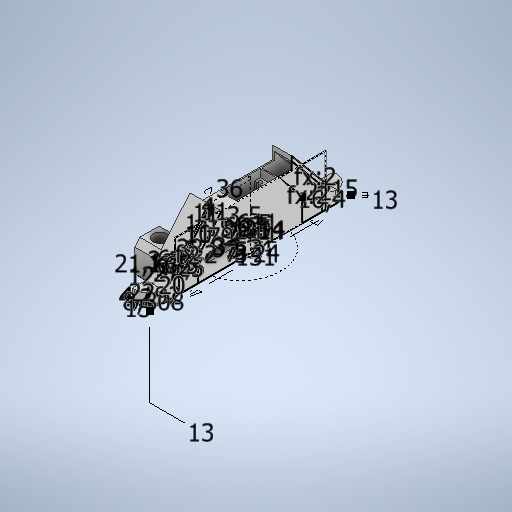
# Autodesk Inventor part: new_back_part
Saved by Autodesk Inventor 2025 (Build 290162000, 162)
## iProperties
Created: 2026-09-04
Part Number: new_back_part
Material: Типовые
Document SubType Name: Modeling
Designer: garin
Density: 1 g/cm^3
Appearance: По умолчанию
Author: garin
Autodesk Inventor part; units mm, degrees
ref_plane "YZ Plane" through (0, 0, 0) normal (1, 0, 0) x (0, 1, 0)
ref_plane "XZ Plane" through (0, 0, 0) normal (0, 1, 0) x (-1, 0, 0)
ref_plane "XY Plane" through (0, 0, 0) normal (0, 0, 1) x (1, 0, 0)
sketch "Эскиз1" plane through (0, 0, 0) normal (0, 1, 0) x (-1, 0, 0)
  line L0 (7, 5) -> (-7, 5)
  line L1 (-7, 5) -> (-7, -19)
  line L2 (-7, -19) -> (7, -19)
  line L3 (7, -19) -> (7, 5)
  line L4 (0, 5) -> (0, 0) construction
  line L5 (-3.5, 3.25) -> (3.5, 3.25) construction
  line L6 (3.5, 3.25) -> (3.5, 6.75) construction
  line L7 (3.5, 6.75) -> (-3.5, 6.75) construction
  line L8 (-3.5, 6.75) -> (-3.5, 3.25) construction
  line L9 (-3.5, 3.25) -> (3.5, 6.75) construction
  line L10 (3.5, 3.25) -> (-3.5, 6.75) construction
  circle A0 centre (3.5, 6.75) radius 1.5
  circle A1 centre (-3.5, 6.75) radius 1.5
  line L11 (2, 6.75) -> (2, 5)
  line L12 (5, 6.75) -> (5, 5)
  line L13 (-2, 6.75) -> (-2, 5)
  line L14 (-5, 6.75) -> (-5, 5)
  line L15 (7, -7) -> (-7, -7) construction
  circle A2 centre (3.5, -20.75) radius 1.5
  circle A3 centre (-3.5, -20.75) radius 1.5
  line L16 (2, -20.75) -> (2, -19)
  line L17 (5, -20.75) -> (5, -19)
  line L18 (-2, -20.75) -> (-2, -19)
  line L19 (-5, -20.75) -> (-5, -19)
  line L20 (0, 0) -> (-8.2, 0) construction
  line L21 (8.2, 65.5) -> (-8.2, 65.5)
  line L22 (-8.2, 65.5) -> (-8.2, -65.5)
  line L23 (-8.2, -65.5) -> (8.2, -65.5)
  line L24 (8.2, -65.5) -> (8.2, 65.5)
  line L25 (-8.2, -65.5) -> (6.8, -65.5)
  line L26 (6.8, -65.5) -> (6.8, -87.5)
  line L27 (6.8, -87.5) -> (4.8, -87.5)
  line L28 (-8.2, -74.5) -> (-8.2, -65.5)
  line L29 (-8.2, 65.5) -> (6.8, 65.5)
  line L30 (6.8, 65.5) -> (6.8, 87.5)
  line L31 (6.8, 87.5) -> (4.8, 87.5)
  line L32 (-8.2, 74.5) -> (-8.2, 65.5)
  arc A4 (4.8, 87.5) -> (-8.2, 74.5) centre (4.8, 74.5) ccw
  arc A5 (-8.2, -74.5) -> (4.8, -87.5) centre (4.8, -74.5) ccw
  circle A6 centre (0, 0) radius 35 construction
  line L33 (24, -5.5) -> (35, -5.5) construction
  line L34 (35, -5.5) -> (35, 5.5) construction
  line L35 (35, 5.5) -> (24, 5.5) construction
  line L36 (24, 5.5) -> (24, -5.5) construction
  line L37 (24, -5.5) -> (34, -5.5) construction
  line L38 (34, -5.5) -> (34, 5.5) construction
  line L39 (34, 5.5) -> (24, 5.5) construction
  line L40 (24, 5.5) -> (24, -5.5) construction
  line L41 (0, 0) -> (35, 0) construction
  line L42 (-5.5, -35) -> (5.5, -35) construction
  line L43 (5.5, -35) -> (5.5, -24) construction
  line L44 (5.5, -24) -> (-5.5, -24) construction
  line L45 (-5.5, -24) -> (-5.5, -35) construction
  line L46 (0, 0) -> (0, -35) construction
  line L47 (7, 10) -> (-7, 10)
  line L48 (-7, 10) -> (-7, -24)
  line L49 (-7, -24) -> (7, -24)
  line L50 (7, -24) -> (7, 10)
  line L51 (7, 10) -> (-7, -24) construction
  line L52 (-7, 10) -> (7, -24) construction
  line L53 (-8.2, 74.5) -> (0.608, 74.5) construction
  line L54 (0.608, 74.5) -> (0.608, 78.692) construction
  line L55 (0.608, 78.692) -> (-8.2, 78.692) construction
  line L56 (-8.2, 78.692) -> (-8.2, 74.5) construction
  circle A7 centre (0.608, 78.692) radius 2.1
  circle A8 centre (0.608, -78.692) radius 2.1
  line L57 (8.2, 0) -> (14.7, 0) construction
  line L58 (14.7, 0) -> (14.7, -19.2) construction
  line L59 (14.7, -19.2) -> (8.2, -19.2) construction
  line L60 (8.2, -19.2) -> (8.2, 0) construction
  circle A9 centre (14.7, -19.2) radius 1.75
  line L61 (8.2, 0) -> (14.7, 0) construction
  line L62 (14.7, 0) -> (14.7, 38.8) construction
  line L63 (14.7, 38.8) -> (8.2, 38.8) construction
  line L64 (8.2, 38.8) -> (8.2, 0) construction
  circle A10 centre (14.7, 38.8) radius 1.75
  line L65 (17.95, -22.45) -> (11.45, -22.45)
  line L66 (11.45, -22.45) -> (11.45, -15.95)
  line L67 (11.45, -15.95) -> (17.95, -15.95)
  line L68 (17.95, -15.95) -> (17.95, -22.45)
  line L69 (17.95, -22.45) -> (11.45, -15.95) construction
  line L70 (11.45, -22.45) -> (17.95, -15.95) construction
  line L71 (11.45, -22.45) -> (8.2, -22.45)
  line L72 (8.2, -22.45) -> (8.2, -15.95)
  line L73 (8.2, -15.95) -> (11.45, -15.95)
  line L74 (11.45, -15.95) -> (11.45, -22.45)
  line L75 (11.45, 35.55) -> (17.95, 35.55)
  line L76 (17.95, 35.55) -> (17.95, 42.05)
  line L77 (17.95, 42.05) -> (11.45, 42.05)
  line L78 (11.45, 42.05) -> (11.45, 35.55)
  line L79 (11.45, 35.55) -> (17.95, 42.05) construction
  line L80 (17.95, 35.55) -> (11.45, 42.05) construction
  line L81 (11.45, 35.55) -> (8.2, 35.55)
  line L82 (8.2, 35.55) -> (8.2, 42.05)
  line L83 (8.2, 42.05) -> (11.45, 42.05)
  line L84 (11.45, 42.05) -> (11.45, 35.55)
  line L85 (8.2, 65.5) -> (26.7, 65.5)
  line L86 (26.7, 65.5) -> (26.7, 44.35)
  line L87 (26.7, 44.35) -> (8.2, 44.35)
  line L88 (8.2, 44.35) -> (8.2, 65.5)
  line L89 (26.7, 54.925) -> (8.2, 54.925) construction
  line L90 (17.45, 65.5) -> (17.45, 44.35) construction
  line L91 (17.95, 42.05) -> (8.2, 42.05)
  line L92 (8.2, 42.05) -> (8.2, 44.35)
  line L93 (8.2, 44.35) -> (17.95, 44.35)
  line L94 (17.95, 44.35) -> (17.95, 42.05)
  line L95 (17.45, 54.925) -> (17.45, 52.925) construction
  circle A11 centre (17.45, 52.925) radius 6
  point P0 (-8.2, -87.5)
  point P1 (-8.2, 87.5)
  point P2 (6.8, -65.5)
  point P3 (6.8, 65.5)
  point P4 (0, -7)
  point P5 (7, 5)
  point P6 (-7, 5)
  point P7 (-7, -19)
  point P8 (8.2, 42.05)
  point P9 (8.2, 35.55)
  point P10 (8.2, -15.95)
  point P11 (8.2, -22.45)
  point P12 (17.95, 44.35)
  point P13 (8.2, 44.35)
  dimension "d0" = 14
  dimension "d1" = 24
  dimension "d2" = 5
  dimension "d3" = 7
  dimension "d4" = 3.5
  dimension "d5" = 3
  dimension "d6" = 3
  dimension "d7" = 8.2
  dimension "d8" = 16.4
  dimension "d9" = 131
  dimension "d10" = 15
  dimension "d11" = 22
  dimension "d12" = 15
  dimension "d13" = 22
  dimension "d14" = 13
  dimension "d15" = 13
  dimension "d24" = 70
  dimension "d25" = 11
  dimension "d26" = 11
  dimension "d27" = 10
  dimension "d28" = 11
  dimension "d29" = 11
  dimension "d32" = 14
  dimension "d33" = 34
  dimension "d77" = 8.808
  dimension "d78" = 4.192
  dimension "d79" = 4.2
  dimension "d82" = 6.5
  dimension "d83" = 19.2
  dimension "d84" = 3.5
  dimension "d85" = 6.5
  dimension "d86" = 38.8
  dimension "d87" = 3.5
  dimension "d88" = 6.5
  dimension "d89" = 6.5
  dimension "d90" = 3.25
  dimension "d91" = 6.5
  dimension "d92" = 6.5
  dimension "d93" = 6.5
  dimension "d94" = 3.25
  dimension "d95" = 6.5
  dimension "d105" = 18.5
  dimension "d106" = 21.15
  dimension "d115" = 2
  dimension "d116" = 12
  constraints: 192 end point, 36 parallel, 24 perpendicular, 21 midpoint, 18 horizontal, 14 point on circle, 14 point on line, 12 centre point, 11 symmetric about line, 8 coincident, 8 tangent, 2 vertical, 3 other
  measures "d0" distance of L2.end L1.end
  measures "d1" distance of L1.end L0.end
  measures "d2" distance of L4.start L4.end
  measures "d3" distance of L7.end L6.end
  measures "d4" distance of L6.end L5.end
  measures "d5" diameter of A0
  measures "d6" diameter of A1
  measures "d7" distance of L20.end L4.end
  measures "d8" distance of L23.end L22.end
  measures "d9" distance of L22.end L21.end
  measures "d10" distance of L26.end point (-8.2, -87.5)
  measures "d11" distance of L25.end L26.end
  measures "d12" distance of point (-8.2, 87.5) L30.end
  measures "d13" distance of L30.end L29.end
  measures "d14" radius of A4
  measures "d15" radius of A5
  measures "d24" diameter of A6
  measures "d25" distance of L35.end L34.end
  measures "d26" distance of L34.end L33.end
  measures "d27" distance of L39.end L38.end
  measures "d28" distance of L44.end L43.end
  measures "d29" distance of L43.end L42.end
  measures "d32" distance of L49.end L48.end
  measures "d33" distance of L48.end L47.end
  measures "d77" distance of L55.end L54.end
  measures "d78" distance of L54.end L53.end
  measures "d79" diameter of A7
  measures "d82" distance of L58.end L59.end
  measures "d83" distance of L57.end L58.end
  measures "d84" diameter of A9
  measures "d85" distance of L63.end L62.end
  measures "d86" distance of L62.end L61.end
  measures "d87" diameter of A10
  measures "d88" distance of L66.end L67.end
  measures "d89" distance of L65.end L66.end
  measures "d90" distance of L72.end L73.end
  measures "d91" distance of L71.end L72.end
  measures "d92" distance of L77.end L76.end
  measures "d93" distance of L76.end L75.end
  measures "d94" distance of L82.end L83.end
  measures "d95" distance of L81.end L82.end
  measures "d105" distance of L86.end L87.end
  measures "d106" distance of L85.end L86.end
  measures "d115" distance of L95.start L95.end
  measures "d116" diameter of A11
extrude "Выдавливание1" add sketch "Эскиз1" along normal blind 44.3 contours L3 L2 L1 L0 | L0 L12 A0 L11 L13 A1 L14 L48 L47 L50 | L0 L11 A0 L12 | L50 L49 L48 L2 L19 A3 L18 L16 A2 L17 | A0 | L17 A2 L16 L2 | L0 L14 A1 L13 | A2 | A1 | L18 A3 L19 L2 | A3 | L24 L23 L22 L21
extrude "Выдавливание2" add sketch "Эскиз1" along normal blind 10 contours L21 L32 A4 L31 L30 | L23 L26 L27 A5 L28 | A7 | A8
extrude "Выдавливание6" cut sketch "Эскиз1" against normal blind 7 from surface at 44.3 contours L3 L2 L1 L0 | L0 L12 A0 L11 L13 A1 L14 L48 L47 L50 | L0 L11 A0 L12 | L50 L49 L48 L2 L19 A3 L18 L16 A2 L17 | A0 | L17 A2 L16 L2 | L0 L14 A1 L13 | A2 | A1 | L18 A3 L19 L2 | A3
extrude "Выдавливание7" cut sketch "Эскиз1" against normal blind 22 from surface at 37.3 contours L3 L2 L1 L0
extrude "Выдавливание8" cut sketch "Эскиз1" against normal blind 6 from surface at 37.3 contours L0 L11 A0 L12 | A0 | L17 A2 L16 L2 | L0 L14 A1 L13 | A2 | A1 | L18 A3 L19 L2 | A3
fillet "Сопряжение1" radius 10 2 edges at (0.7, 10, 65.5) (0.7, 10, -65.5)
sketch "Эскиз4" plane through (8.2, 44.3, 65.5) normal (1, 0, 0) x (0, 0, -1)
  line L0 (131, 0) -> (0, 0) construction
  line L1 (131, -44.3) -> (0, -44.3) construction
  line L2 (0, 0) -> (131, 0) construction
  line L3 (131, 0) -> (131, -44.3) construction
  line L4 (131, -44.3) -> (0, -44.3) construction
  line L5 (0, -44.3) -> (0, 0) construction
  line L6 (65.5, 0) -> (65.5, -44.3) construction
  line L7 (65.5, 0) -> (29.5, 0) construction
  line L8 (29.5, 0) -> (29.5, 11)
  line L9 (29.5, 11) -> (65.5, 11) construction
  line L10 (65.5, 11) -> (65.5, 0) construction
  line L11 (0, -44.3) -> (0, -24.3)
  line L12 (0, -24.3) -> (29.5, 11)
  line L13 (29.5, 0) -> (40.5, 0)
  line L14 (40.5, 0) -> (21.4751, -22.7653)
  line L15 (0, -24.3) -> (20.1926, -24.3) construction
  line L16 (20.1926, -26.3) -> (20.1926, -44.3)
  line L17 (0, -44.3) -> (20.1926, -44.3) construction
  line L18 (29.5, 11) -> (29.5, 7) construction
  line L19 (29.5, 7) -> (3.3428, -24.3)
  line L20 (3.3428, -24.3) -> (3.3428, -44.3)
  line L21 (0, -44.3) -> (20.1926, -44.3)
  line L22 (101.5, 0) -> (101.5, 11)
  line L23 (131, -44.3) -> (131, -24.3)
  line L24 (131, -24.3) -> (101.5, 11)
  line L25 (101.5, 0) -> (90.5, 0)
  line L26 (90.5, 0) -> (109.5249, -22.7653)
  line L27 (110.8074, -26.3) -> (110.8074, -44.3)
  line L28 (101.5, 7) -> (127.6572, -24.3)
  line L29 (127.6572, -24.3) -> (127.6572, -44.3)
  line L30 (131, -44.3) -> (110.8074, -44.3)
  line L31 (20.3074, 0) -> (0, 0)
  line L32 (0, 0) -> (0, -24.3)
  line L33 (110.6926, 0) -> (131, 0)
  line L34 (131, 0) -> (131, -24.3)
  line L35 (21.4751, -22.7653) -> (20.1926, -26.3)
  line L36 (109.5249, -22.7653) -> (110.8074, -26.3)
  point P0 (3.3428, -44.3)
  point P1 (110.8074, -24.3)
  point P2 (127.6572, -44.3)
  point P3 (110.6926, 0)
  dimension "d54" = 36
  dimension "d55" = 11
  dimension "d56" = 20
  dimension "d57" = 11
  dimension "d58" = 4
  dimension "d73" = 2
  dimension "d74" = 2
  dimension "d75" = 2
  dimension "d76" = 2
  constraints: 70 end point, 15 point on line, 11 symmetric about line, 6 parallel, 5 perpendicular, 4 collinear, 2 horizontal, 1 midpoint, 1 vertical
  measures "d54" distance of L8.end L9.end
  measures "d55" distance of L7.end L8.end
  measures "d56" distance of L4.end L11.end
  measures "d57" distance of L7.end L13.end
  measures "d58" distance of L8.end L18.end
  measures "d73" distance of L14.end L15.end
  measures "d74" distance of L16.start L15.end
  measures "d75" distance of L26.end point (110.807, -24.3)
  measures "d76" distance of L27.start point (110.807, -24.3)
ref_plane "РабПлоскость1" through (7, 44.3, 65.5) normal (1, 0, 0) x (0, 0, -1)
ref_plane "РабПлоскость2" through (-7, 0, -65.5) normal (-1, 0, 0) x (0, 0, 1)
extrude "Выдавливание9" cut sketch "Эскиз4" against normal blind 14 from surface at -1.2 contours L13 L14 L35 L16 L21 L20 L19 L8 | L22 L28 L29 L30 L27 L36 L26 L25 | L22 L24 L23 L30 L29 L28
extrude "Выдавливание10" add sketch "Эскиз4" against normal blind 16.4 contours L19 L20 L21 L11 L12 L8 | L22 L24 L23 L30 L29 L28
extrude "Выдавливание11" cut sketch "Эскиз4" against normal blind 16.4 contours L12 L32 L31 | L33 L34 L24
extrude "Выдавливание12" add sketch "Эскиз4" against normal blind 1.2 contours L13 L14 L35 L16 L21 L20 L19 L8 | L22 L28 L29 L30 L27 L36 L26 L25 | L22 L24 L23 L30 L29 L28
extrude "Выдавливание13" add sketch "Эскиз4" along normal blind 1.2 from surface at -16.4 contours L13 L14 L35 L16 L21 L20 L19 L8 | L22 L28 L29 L30 L27 L36 L26 L25 | L22 L24 L23 L30 L29 L28
fillet "Сопряжение2" radius 2 2 edges at (-6.8, 10, 65.5) (-6.8, 10, -65.5)
fillet "Сопряжение3" radius 1 1 edges at (0, 44.3, 10)
extrude "Выдавливание14" cut sketch "Эскиз1" along normal blind 6 contours A7 | A8
extrude "Выдавливание15" add sketch "Эскиз1" along normal blind 11.6 contours L87 L94 L77 L83 L24 | L83 L78 L81 L24 | L77 L76 L75 L78 | L73 L66 L71 L24 | L67 L68 L65 L66 | A9 | A10
fillet "Сопряжение4" radius 2 6 edges at (-17.95, 5.8, -22.45) (-8.2, 5.8, -22.45) (-8.2, 5.8, -15.95) (-17.95, 5.8, -15.95) (-17.95, 5.8, 35.55) (-8.2, 5.8, 35.55)
extrude "Выдавливание16" cut sketch "Эскиз1" against normal blind 6 from surface at 11.6 contours A9 | A10
sketch "Эскиз6" plane through (-8.2, 44.3, 36) normal (-1, 0, 0) x (0, 0, 1)
  line L0 (0.6, -29.4) -> (0.6, -28.84) projected
  arc A0 (-0.7, -30.7) -> (0.6, -29.4) centre (-0.7, -29.4) ccw projected
  line L1 (-0.7, -30.7) -> (-7.04, -30.7) projected
  arc A1 (-8.34, -29.4) -> (-7.04, -30.7) centre (-7.04, -29.4) ccw projected
  line L2 (-8.34, -29.4) -> (-8.34, -28.84) projected
  arc A2 (-7.04, -27.54) -> (-8.34, -28.84) centre (-7.04, -28.84) ccw projected
  line L3 (-0.7, -27.54) -> (-7.04, -27.54) projected
  arc A3 (0.6, -28.84) -> (-0.7, -27.54) centre (-0.7, -28.84) ccw projected
  arc A4 (-7.04, -27.84) -> (-8.04, -28.84) centre (-7.04, -28.84) ccw projected
  line L4 (-8.04, -29.4) -> (-8.04, -28.84) projected
  arc A5 (-8.04, -29.4) -> (-7.04, -30.4) centre (-7.04, -29.4) ccw projected
  line L5 (-7.04, -30.4) -> (-0.7, -30.4) projected
  arc A6 (-0.7, -30.4) -> (0.3, -29.4) centre (-0.7, -29.4) ccw projected
  line L6 (0.3, -28.84) -> (0.3, -29.4) projected
  arc A7 (0.3, -28.84) -> (-0.7, -27.84) centre (-0.7, -28.84) ccw projected
  line L7 (-0.7, -27.84) -> (-7.04, -27.84) projected
  arc A8 (-7.04, -25.54) -> (-10.34, -28.84) centre (-7.04, -28.84) ccw construction
  line L8 (-10.34, -28.84) -> (-10.34, -29.4) construction
  arc A9 (-10.34, -29.4) -> (-7.04, -32.7) centre (-7.04, -29.4) ccw construction
  line L9 (-7.04, -32.7) -> (-0.7, -32.7) construction
  arc A10 (-0.7, -32.7) -> (2.6, -29.4) centre (-0.7, -29.4) ccw
  line L10 (2.6, -29.4) -> (2.6, -28.84)
  arc A11 (2.6, -28.84) -> (-0.7, -25.54) centre (-0.7, -28.84) ccw
  line L11 (-0.7, -25.54) -> (-7.04, -25.54) construction
  line L12 (-15.7, -27.8) -> (-21.3, -27.8) projected
  arc A12 (-15.25, -28.25) -> (-15.7, -27.8) centre (-15.7, -28.25) ccw projected
  line L13 (-15.25, -29.5702) -> (-15.25, -28.25) projected
  arc A13 (-15.3734, -29.8798) -> (-15.25, -29.5702) centre (-15.7, -29.5702) ccw projected
  line L14 (-16.0179, -30.5596) -> (-15.3734, -29.8798) projected
  arc A14 (-16.3445, -30.7) -> (-16.0179, -30.5596) centre (-16.3445, -30.25) ccw projected
  line L15 (-18.34, -30.7) -> (-16.3445, -30.7) projected
  line L16 (-20.6555, -30.7) -> (-18.66, -30.7) projected
  arc A15 (-20.9821, -30.5596) -> (-20.6555, -30.7) centre (-20.6555, -30.25) ccw projected
  line L17 (-21.6266, -29.8798) -> (-20.9821, -30.5596) projected
  arc A16 (-21.75, -29.5702) -> (-21.6266, -29.8798) centre (-21.3, -29.5702) ccw projected
  line L18 (-21.75, -28.25) -> (-21.75, -29.5702) projected
  arc A17 (-21.3, -27.8) -> (-21.75, -28.25) centre (-21.3, -28.25) ccw projected
  line L19 (-15.25, -28.9101) -> (-8.34, -28.9101) construction
  line L20 (-11.795, -28.9101) -> (-11.795, -27.9101) construction
  arc A18 (-26.19, -29.4) -> (-22.89, -32.7) centre (-22.89, -29.4) ccw
  line L21 (-26.19, -29.4) -> (-26.19, -28.84)
  arc A19 (-22.89, -25.54) -> (-26.19, -28.84) centre (-22.89, -28.84) ccw
  line L22 (-0.7, -25.54) -> (-22.89, -25.54)
  line L23 (-22.89, -32.7) -> (-0.7, -32.7)
  point P0 (-36, -44.3)
  dimension "d101" = 2
  dimension "d102" = 1
  constraints: 18 end point, 12 point on circle, 6 centre point, 6 symmetric about line, 2 midpoint, 2 perpendicular, 1 collinear, 1 parallel, 1 point on line, 1 tangent, 9 other
  measures "d101" distance between parallel lines of L3 L11
  measures "d102" distance of L20.start L20.end
extrude "Выдавливание17" cut sketch "Эскиз6" against normal blind 16.4 contours A0 L1 A1 L2 A2 L3 A3 L0 | L7 A7 L6 A6 L5 A5 L4 A4 | L23 A18 L21 A19 L22 A11 L10 A10
extrude "Выдавливание18" add sketch "Эскиз1" along normal blind 25.2 contours L85 L86 L87 L24 | A11
extrude "Выдавливание19" cut sketch "Эскиз4" against normal blind 35 contours L12 L32 L31
extrude "Выдавливание20" cut sketch "Эскиз1" against normal blind 24 from surface at 25.2 contours A11
fillet "Сопряжение5" radius 2 1 edges at (-17.95, 5.8, 44.35)
equation "\"d74\" = d73"
equation "\"d75\" = d73"
equation "\"d76\" = d75"
